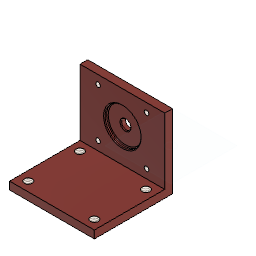
SoporteNEMA17 v10 v4 (Autodesk Fusion 360 design; units mm, degrees)
Autodesk Fusion 360 part; units mm, degrees
sketch "Sketch1" plane through (0, 0, 0) normal (0, 0, 1) x (1, 0, 0)
  line L0 (21.125, 21.125) -> (-21.125, 21.125)
  line L1 (-21.125, 21.125) -> (-21.125, -21.125)
  line L2 (-21.125, -21.125) -> (21.125, -21.125)
  line L3 (21.125, -21.125) -> (21.125, 21.125)
  line L4 (21.125, 21.125) -> (-21.125, -21.125) construction
  line L5 (-21.125, 21.125) -> (21.125, -21.125) construction
  dimension "d1" = 42.25
  dimension "d2" = 42.25
  constraint horizontal L0
  constraint perpendicular L0 L1
  constraint parallel L0 L2
  constraint parallel L1 L3
  constraint coincident L4 origin
  constraint coincident L5 origin
  measures "d1" distance of L1.end L2.end
  measures "d2" distance of L0.end L1.end
extrude "Extrude1" add sketch "Sketch1" along normal blind 5
sketch "Sketch2" plane through (0, 0, 5) normal (0, 0, 1) x (-1, 0, 0)
  line L0 (-21.125, 21.125) -> (-21.125, -21.125)
  line L1 (-21.125, -21.125) -> (21.125, -21.125)
  line L2 (21.125, -21.125) -> (21.125, 21.125)
  line L3 (21.125, 21.125) -> (-21.125, 21.125)
  circle A0 centre (0, 0) radius 11.5
  line L4 (-21.125, 0) -> (21.125, 0) construction
  line L5 (0, -21.125) -> (0, 21.125) construction
  point P0 (-15.5, -15.5)
  point P1 (15.5, -15.5)
  point P2 (-15.5, 15.5)
  point P3 (15.5, 15.5)
  dimension "d5" = 23
  dimension "d32" = 5.625
  dimension "d33" = 5.625
  constraint coincident A0.centre origin
  constraint midpoint L0 L4.start
  constraint midpoint L2 L4.end
  constraint midpoint L1 L5.start
  constraint midpoint L3 L5.end
  constraint symmetric P0 L5 P1
  constraint symmetric P0 L4 P2
  constraint symmetric L4 P1 P3
  measures "d5" diameter of A0
  measures "d32" distance of L0 P0
  measures "d33" distance of L1 P0
extrude "Extrude2" cut sketch "Sketch2" against normal blind 2 contours A0
sketch "Sketch3" plane through (0, 0, 3) normal (0, 0, 1) x (-1, 0, 0)
  circle A0 centre (0, 0) radius 11.5
  circle A1 centre (0, 0) radius 3
  dimension "d8" = 6
  constraint coincident A0.centre A1.centre
  measures "d8" diameter of A1
extrude "Extrude3" cut sketch "Sketch3" against normal blind 3 contours A1
sketch "Sketch6" plane through (0, 0, 0) normal (0, 0, -1) x (1, 0, 0)
  circle A0 centre (0, 0) radius 3
  line L0 (21.125, -21.125) -> (21.125, 21.125)
  line L1 (21.125, 21.125) -> (-21.125, 21.125)
  line L2 (-21.125, 21.125) -> (-21.125, -21.125)
  line L3 (-21.125, -21.125) -> (21.125, -21.125)
extrude "Extrude4" add 1 faces at (-7.0417, -21.125, 1.6667) along direction (0, -1, 0) blind 5
sketch "Sketch5" plane through (0, 0, 5) normal (0, 0, 1) x (-1, 0, 0)
  circle A0 centre (0, 0) radius 11.5
  line L0 (-21.125, 26.125) -> (-21.125, -21.125)
  line L1 (-21.125, -21.125) -> (21.125, -21.125)
  line L2 (21.125, -21.125) -> (21.125, 26.125)
  line L3 (21.125, 26.125) -> (-21.125, 26.125)
  line L4 (21.125, 23.625) -> (-21.125, 23.625)
  line L5 (21.125, -21.125) -> (-21.125, -21.125)
  line L6 (-21.125, -21.125) -> (-21.125, 21.125)
  dimension "d15" = 2.5
  constraint coincident L2 L4.start
  constraint coincident L0 L4.end
  constraint perpendicular L0 L4
  measures "d15" distance of L3 L4
extrude "Extrude5" add sketch "Sketch5" along normal blind 34 contours L0 L2 L3 L4
fillet "Fillet1" radius 0.5 2 faces at (-8.6127, 0.7204, 3) (-11.4857, 0.5732, 3.6667)
sketch "Sketch11" plane through (0, 0, 0) normal (0, 0, -1) x (1, 0, 0)
  line L0 (0, -0.125) -> (0, -42.125) construction
  line L1 (21.1283, 0) -> (-21.125, 0) construction
  line L2 (21.125, -21.125) -> (21.125, 21.125)
  line L3 (-21.125, -21.125) -> (21.125, -21.125)
  line L4 (-21.125, 21.125) -> (-21.125, -21.125)
  constraint vertical L0
  constraint perpendicular L0 L1
  constraint midpoint L0 L3
  constraint midpoint L1.end L4
hole "Hole2" at (15.5, 15.5, 0) at (-15.5, 15.5, 0) at (-15.5, -15.5, 0) at (15.5, -15.5, 0) direction (0, 0, 1) diameter 3.4 depth 5 tip angle 118 counterbore diameter 6.5 counterbore depth 3
move_body "Move1" bodies 1 to x (1, 0, 0) y (0, 0, 1) z (0, -1, 0) at (0, -26.125, 26.125)
extrude "Extrude6" cut 1 faces at (7.0417, -65.125, 1.6667) along direction (0, 1, 0) blind 6.139
extrude "Extrude7" add 1 faces at (-7.0417, -40.412, 2.5) along direction (0, 0, 1) blind 2.5
sketch "Sketch14" plane through (0, 0, 5) normal (0, 0, 1) x (-1, 0, 0)
  line L0 (21.125, 58.986) -> (-21.125, 58.986)
  line L1 (-21.125, 58.986) -> (-21.125, 31.125)
  line L2 (-21.125, 31.125) -> (21.125, 31.125)
  line L3 (21.125, 31.125) -> (21.125, 58.986)
  line L4 (-21.125, 45.0555) -> (21.125, 45.0555) construction
  line L5 (0, 58.986) -> (0, 31.125) construction
  circle A0 centre (17.125, 35.125) radius 1.5
  circle A1 centre (17.125, 54.986) radius 1.5
  circle A2 centre (-17.125, 35.125) radius 1.5
  circle A3 centre (-17.125, 54.986) radius 1.5
  dimension "d82" = 3
  dimension "d83" = 4
  dimension "d84" = 4
  dimension "d85" = 3
  dimension "d86" = 4
  dimension "d87" = 4
  dimension "d88" = 3
  dimension "d89" = 3
  dimension "d90" = 4
  dimension "d91" = 4
  dimension "d92" = 4
  dimension "d93" = 4
  constraint midpoint L1 L4.start
  constraint midpoint L3 L4.end
  constraint midpoint L0 L5.start
  constraint midpoint L2 L5.end
  measures "d82" diameter of A0
  measures "d83" distance of L2 A0.centre
  measures "d84" distance of L3 A0.centre
  measures "d85" diameter of A1
  measures "d86" distance of L3 A1.centre
  measures "d87" distance of L0 A1.centre
  measures "d88" diameter of A2
  measures "d89" diameter of A3
  measures "d90" distance of L1 A2.centre
  measures "d91" distance of L2 A2.centre
  measures "d92" distance of L1 A3.centre
  measures "d93" distance of L0 A3.centre
extrude "Extruir14" add 1 faces at (-21.125, -27.7917, 17.4167) along direction (-1, 0, 0) blind 6
extrude "Extruir15" add 1 faces at (21.125, -27.7917, 17.4167) along direction (1, 0, 0) blind 6
extrude "Extruir16" add 1 faces at (-9.0417, -58.986, 3.3333) along direction (0, -1, 0) blind 17.169
sketch "Boceto17" plane through (0, 0, 5) normal (0, 0, 1) x (-1, 0, 0)
  line L0 (-27.125, 76.155) -> (-27.125, 31.125)
  line L1 (-27.125, 31.125) -> (27.125, 31.125)
  line L2 (27.125, 31.125) -> (27.125, 76.155)
  line L3 (27.125, 76.155) -> (-27.125, 76.155)
  circle A0 centre (21.125, 37.125) radius 3
  circle A1 centre (-21.125, 37.125) radius 3
  circle A2 centre (21.125, 70.155) radius 3
  circle A3 centre (-21.125, 70.155) radius 3
  point P0 (22.3785, 34.6118)
  dimension "d100" = 6
  dimension "d101" = 6
  dimension "d102" = 6
  dimension "d103" = 6
  dimension "d104" = 6
  dimension "d105" = 6
  dimension "d106" = 6
  dimension "d107" = 6
  dimension "d108" = 6
  dimension "d109" = 6
  dimension "d110" = 6
  dimension "d111" = 6
  measures "d100" diameter of A0
  measures "d101" distance of L2 A0.centre
  measures "d102" distance of L1 A0.centre
  measures "d103" diameter of A1
  measures "d104" distance of L1 A1.centre
  measures "d105" distance of L0 A1.centre
  measures "d106" diameter of A2
  measures "d107" diameter of A3
  measures "d108" distance of L2 A2.centre
  measures "d109" distance of L3 A2.centre
  measures "d110" distance of L0 A3.centre
  measures "d111" distance of L3 A3.centre
thread "Rosca5" "ISO Metric profile 3.5 M3.5x0.6 M3.5x0.6 6H" major diameter 3.5995 minor diameter 2.93 pitch 0.6 angle 60 resizes the face on face at (-15.3307, -30.4583, 43.3166)
thread "Rosca6" "ISO Metric profile 3.5 M3.5x0.6 M3.5x0.6 6H" major diameter 3.5995 minor diameter 2.93 pitch 0.6 angle 60 resizes the face on face at (15.5847, -29.7917, 43.3229)
thread "Rosca7" "ISO Metric profile 3.5 M3.5x0.6 M3.5x0.6 6H" major diameter 3.5995 minor diameter 2.93 pitch 0.6 angle 60 resizes the face on face at (-15.4153, -29.7917, 12.3229)
thread "Rosca8" "ISO Metric profile 3.5 M3.5x0.6 M3.5x0.6 6H" major diameter 3.5995 minor diameter 2.93 pitch 0.6 angle 60 resizes the face on face at (15.5847, -29.7917, 12.3229)
extrude "Extruir18" cut sketch "Boceto17" against normal blind 29 contours A0 | A1 | A2 | A3
thread "Rosca9" "ISO Metric profile 6.0 M6x1 M6x1 6H" major diameter 6.147 minor diameter 5.035 pitch 1 angle 60 resizes the face on face at (-18.1399, -36.8263, 1.6667)
thread "Rosca10" "ISO Metric profile 6.0 M6x1 M6x1 6H" major diameter 6.147 minor diameter 5.035 pitch 1 angle 60 resizes the face on face at (24.1101, -36.8263, 1.6667)
thread "Rosca11" "ISO Metric profile 6.0 M6x1 M6x1 6H" major diameter 6.147 minor diameter 5.035 pitch 1 angle 60 resizes the face on face at (-23.6849, -71.7193, 1.6667)
thread "Rosca12" "ISO Metric profile 6.0 M6x1 M6x1 6H" major diameter 6.147 minor diameter 5.035 pitch 1 angle 60 resizes the face on face at (18.5651, -71.7193, 1.6667)
